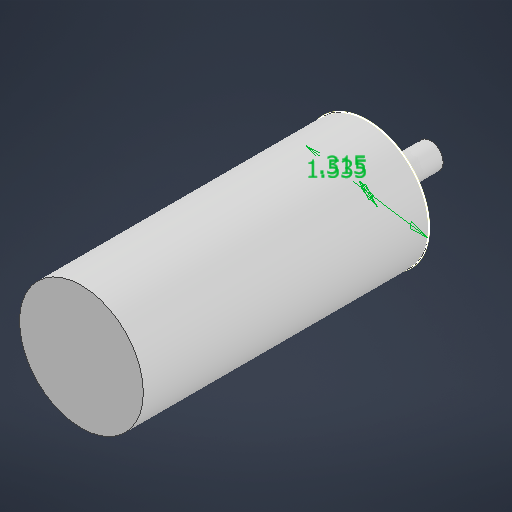
# Autodesk Inventor part: PG36M555_Motor_Dummy
Saved by Autodesk Inventor 2026.2 (Build 302298010, 298A)
## iProperties
Created: 2026-03-25
Part Number: PG36M555_Motor_Dummy
Material: Generic
Document SubType Name: Modeling
Designer: Srishanth Dhondy
Density: 1 g/cm^3
Appearance: Default
Author: Srishanth Dhondy
Autodesk Inventor part; units mm, degrees
ref_plane "YZ Plane" through (0, 0, 0) normal (1, 0, 0) x (0, 1, 0)
ref_plane "XZ Plane" through (0, 0, 0) normal (0, 1, 0) x (-1, 0, 0)
ref_plane "XY Plane" through (0, 0, 0) normal (0, 0, 1) x (1, 0, 0)
sketch "Sketch1" plane through (0, 0, 0) normal (0, 0, 1) x (1, 0, 0)
  circle A0 centre (0, 0) radius 19.5
  circle A1 centre (0, 0) radius 4
  dimension "d0" = 39
  dimension "d3" = 8
  constraints: 2 centre point, 2 coincident
  measures "d0" diameter of A0
  measures "d3" diameter of A1
extrude "Extrusion1" add sketch "Sketch1" along normal blind 90 contours A0 | A1
extrude "Extrusion2" add sketch "Sketch1" against normal blind 20 contours A1
sketch "Sketch2" plane through (0, 0, 0) normal (0, 0, -1) x (-1, 0, 0)
  circle A0 centre (0, 0) radius 4 projected
  circle A1 centre (0, 0) radius 19.5 projected
sketch "Sketch3" plane through (0, 0, 0) normal (0, 0, -1) x (-1, 0, 0)
  circle A0 centre (0, 0) radius 19.5 projected
  circle A1 centre (0, 0) radius 14 construction
  point P0 (14, 0)
  dimension "d6" = 28
  constraints: 1 coincident, 1 horizontal alignment, 2 other
hole "Hole1" at (-14, 0, 0) direction (0, 0, 1) diameter 3 depth 6 tip angle 118
pattern_circular "Circular Pattern1" count 4 over 360 about axis through (0, 0, 0) along (0, 0, 1) of "Hole1"
body "Solid1"
